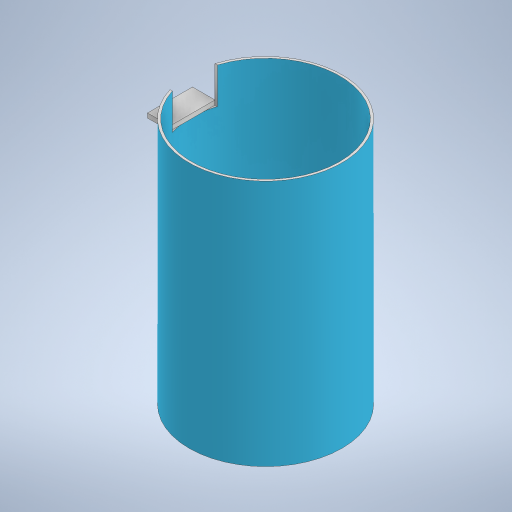
# Autodesk Inventor part: tuvo
Saved by Autodesk Inventor 2023 (Build 270158000, 158)
## iProperties
Created: 2022-04-04
Part Number: tuvo
Material: Genérico
Document SubType Name: Modeling
Designer: isaac
Density: 1 g/cm^3
Appearance: Valor por defecto
Author: isaac
Autodesk Inventor part; units mm, degrees
ref_plane "YZ Plane" through (0, 0, 0) normal (1, 0, 0) x (0, 1, 0)
ref_plane "XZ Plane" through (0, 0, 0) normal (0, 1, 0) x (-1, 0, 0)
ref_plane "XY Plane" through (0, 0, 0) normal (0, 0, 1) x (1, 0, 0)
sketch "Boceto1" plane through (0, 0, 0) normal (0, 1, 0) x (-1, 0, 0)
  circle A0 centre (0, 0) radius 16.5
  circle A1 centre (0, 0) radius 17
  dimension "d0" = 33
  dimension "d1" = 34
  constraints: 2 centre point, 2 coincident
  measures "d0" diameter of A0
  measures "d1" diameter of A1
extrude "Extrusión1" add sketch "Boceto1" along normal blind 55
sketch "Boceto2" plane through (0, 0, 0) normal (1, 0, 0) x (0, 1, 0)
  line L0 (55, 5) -> (47, 5)
  line L1 (47, 5) -> (47, -5)
  line L2 (47, -5) -> (55, -5)
  line L3 (55, -5) -> (55, 5)
  line L4 (55, 16.5) -> (55, -16.5) construction
  line L5 (0, 16.5) -> (0, -16.5) construction
  point P0 (0, 0)
  point P1 (55, 0)
  dimension "d4" = 10
  dimension "d5" = 8
  constraints: 8 end point, 2 parallel, 1 horizontal, 1 horizontal alignment, 1 midpoint, 1 perpendicular, 1 vertical alignment
  measures "d4" distance between parallel lines of L2 L0
  measures "d5" distance between parallel lines of L1 L3
extrude "Extrusión2" cut sketch "Boceto2" against normal blind 55
sketch "Boceto3" plane through (-16.2481, 47, 5) normal (0, 1, 0) x (1, 0, 0)
  arc A0 (0, 10) -> (0, 0) centre (16.2481, 5) ccw construction
  line L0 (0.5239, 0) -> (0, 0) construction
  arc A1 (0.5239, 10) -> (0.5239, 0) centre (16.2481, 5) ccw construction
  line L1 (0.5239, 10) -> (0, 10) construction
  line L2 (0, 10) -> (-5, 10)
  line L3 (-5, 10) -> (-5, 0)
  line L4 (-5, 0) -> (0, 0)
  line L5 (0, 0) -> (0, 10)
  dimension "d8" = 5
  dimension "d9" = 10
  constraints: 8 end point, 2 parallel, 1 horizontal, 1 perpendicular
  measures "d8" distance between parallel lines of L5 L3
  measures "d9" distance between parallel lines of L2 L4
extrude "Extrusión3" add sketch "Boceto3" along normal blind 1
